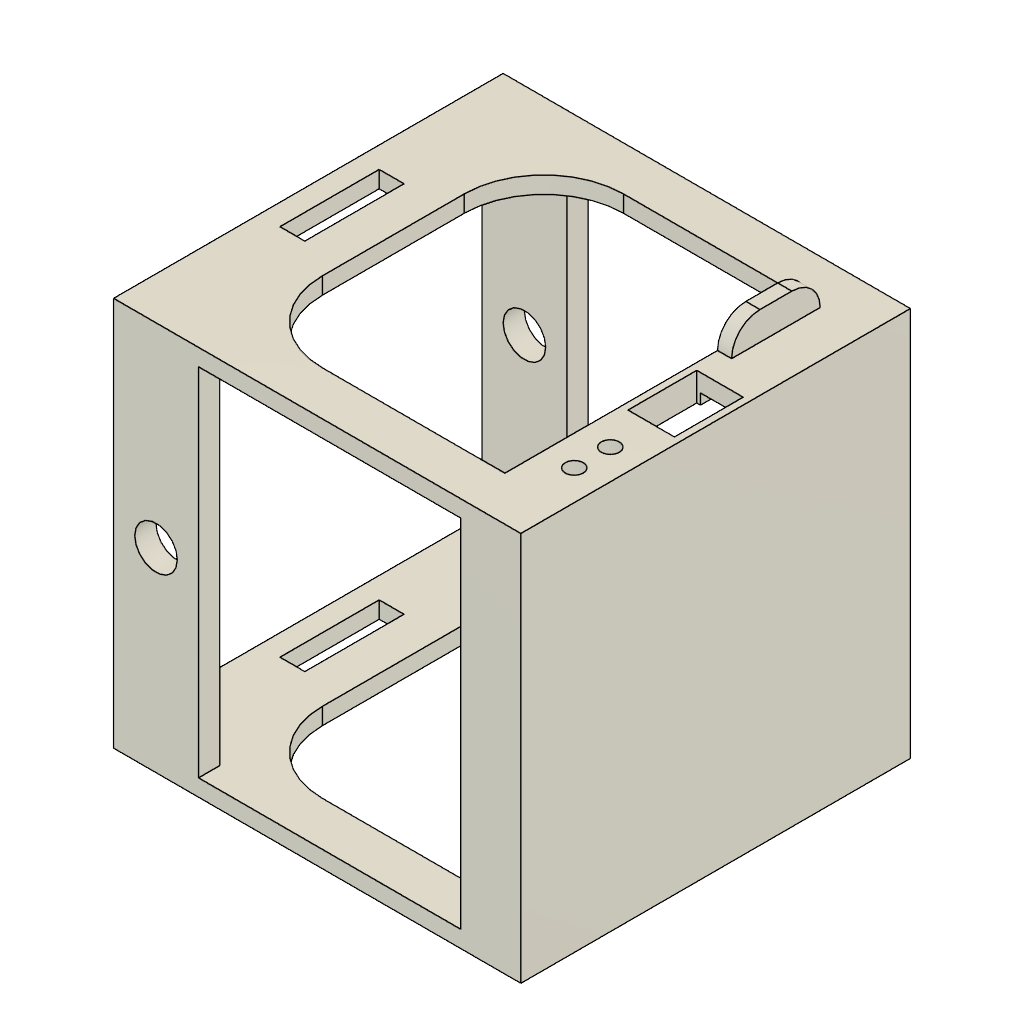
Cansat_D1 (Autodesk Fusion 360 design; units mm, degrees)
part number: 2026-09-08-22-36-42-588
Autodesk Fusion 360 part; units mm, degrees
note: some values were not read from the file. Set by a fixed rule: which sketch regions a step uses.
sketch "Sketch1" plane through (0, 0, 0) normal (0, 1, 0) x (1, 0, 0)
  line L0 (-55, -55) -> (55, -55)
  line L1 (55, -55) -> (55, 55)
  line L2 (55, 55) -> (-55, 55)
  line L3 (-55, 55) -> (-55, -55)
  line L4 (-55, -55) -> (55, 55) construction
  line L5 (55, -55) -> (-55, 55) construction
  line L6 (-50, 50) -> (50, 50)
  line L7 (50, 50) -> (50, -50)
  line L8 (50, -50) -> (-50, -50)
  line L9 (-50, -50) -> (-50, 50)
  line L10 (-50, 50) -> (50, -50) construction
  line L11 (50, 50) -> (-50, -50) construction
  dimension "d1" = 110
  dimension "d2" = 110
  dimension "d3" = 100
  dimension "d4" = 100
  constraint horizontal L0
  constraint perpendicular L0 L1
  constraint parallel L0 L2
  constraint parallel L1 L3
  constraint coincident L4 origin
  constraint coincident L5 origin
  constraint horizontal L6
  constraint perpendicular L6 L7
  constraint parallel L6 L8
  constraint parallel L7 L9
  constraint coincident L10 origin
  constraint coincident L11 origin
  measures "d1" distance of L1.end L2.end
  measures "d2" distance of L0.end L1.end
  measures "d3" distance of L7.end L8.end
  measures "d4" distance of L6.end L7.end
extrude "Extrude1" add sketch "Sketch1" along normal blind 5 contours L6 L7 L8 L9 makes body 1
extrude "Extrude2" add sketch "Sketch1" along normal blind 15 bodies 1
extrude "Extrude3" cut 1 faces at (-16.6667, 5, -16.6667) along direction (0, -1, 0) blind 1 on bodies 1 bodies 1
sketch "Sketch2" plane through (0, 15, 0) normal (0, 1, 0) x (-1, 0, 0)
  line L0 (-50, 50) -> (50, 50)
  line L1 (50, 50) -> (50, -50)
  line L2 (50, -50) -> (-50, -50)
  line L3 (-50, -50) -> (-50, 50)
  line L4 (55, -55) -> (55, 55)
  line L5 (55, 55) -> (-55, 55)
  line L6 (-55, 55) -> (-55, -55)
  line L7 (-55, -55) -> (55, -55)
sketch "Sketch3" plane through (0, 15, 0) normal (0, 1, 0) x (-1, 0, 0)
  line L0 (55, -55) -> (50, -55)
  line L1 (50, -55) -> (50, 55)
  line L2 (50, 55) -> (55, 55)
  line L3 (55, 55) -> (55, -55)
  line L4 (-50, -55) -> (-55, -55)
  line L5 (-55, -55) -> (-55, 55)
  line L6 (-55, 55) -> (-50, 55)
  line L7 (-50, 55) -> (-50, -55)
  constraint horizontal L0
  constraint vertical L1
  constraint horizontal L2
  constraint vertical L3
  constraint horizontal L4
  constraint vertical L5
  constraint horizontal L6
  constraint vertical L7
extrude "Extrude4" add sketch "Sketch3" along normal blind 100 bodies 1
sketch "Sketch4" plane through (55, 0, 0) normal (1, 0, 0) x (0, 0, -1)
  line L0 (-55, 0) -> (55, 0)
  line L1 (55, 0) -> (55, 115)
  line L2 (55, 115) -> (-55, 115)
  line L3 (-55, 115) -> (-55, 0)
  line L4 (0, 115) -> (0, 109)
  line L5 (0, 109) -> (0, 102)
  line L6 (0, 102) -> (0, 105.5)
  line L7 (0, 105.5) -> (55, 105.5)
  line L8 (55, 105.5) -> (49, 105.5)
  line L9 (49, 109) -> (-49, 109)
  line L10 (-49, 109) -> (-49, 102)
  line L11 (-49, 102) -> (49, 102)
  line L12 (49, 102) -> (49, 109)
  line L13 (49, 109) -> (-49, 102) construction
  line L14 (-49, 109) -> (49, 102) construction
  point P0 (0, 105.5)
  dimension "d13" = 98
  dimension "d14" = 7
  constraint midpoint L2 L4.start
  constraint perpendicular L2 L4
  constraint perpendicular L2 L5
  constraint midpoint L5 P0
  constraint coincident L1 L7.end
  constraint perpendicular L1 L7
  constraint coincident L7 L8.end
  constraint horizontal L9
  constraint perpendicular L9 L10
  constraint parallel L9 L11
  constraint parallel L10 L12
  constraint coincident L13 P0
  constraint coincident L14 P0
  constraint coincident P0 L6.end
  measures "d13" distance of L10.end L11.end
  measures "d14" distance of L9.end L10.end
extrude "Extrude5" cut sketch "Sketch4" against normal blind 163 contours L5 L6 L7 L11 L12 | L5 L7 L9 L12 | L5 L6 L9 L10 L11 bodies 1
sketch "Sketch5" plane through (55, 0, 0) normal (1, 0, 0) x (0, 0, -1)
  line L0 (-49, 109) -> (49, 109)
  line L1 (49, 109) -> (49, 102)
  line L2 (49, 102) -> (-49, 102)
  line L3 (-49, 102) -> (-49, 109)
  line L4 (-55, 0) -> (55, 0)
  line L5 (55, 0) -> (55, 115)
  line L6 (55, 115) -> (-55, 115)
  line L7 (-55, 115) -> (-55, 0)
  line L8 (-55, 115) -> (-49, 115)
  line L9 (-49, 115) -> (-49, 109)
  line L10 (-49, 109) -> (-55, 109)
  line L11 (-55, 109) -> (-55, 115)
  line L12 (55, 115) -> (49, 115)
  line L13 (49, 115) -> (49, 109)
  line L14 (49, 109) -> (55, 109)
  line L15 (55, 109) -> (55, 115)
  constraint horizontal L8
  constraint vertical L9
  constraint horizontal L10
  constraint vertical L11
  constraint coincident L0.start L3.end
  constraint coincident L6.end L7.start
  constraint horizontal L12
  constraint vertical L13
  constraint horizontal L14
  constraint vertical L15
  constraint coincident L0.end L1.start
  constraint coincident L5.end L6.start
extrude "Extrude6" add sketch "Sketch5" against normal blind 110 separate body contours L6 L7 L8 L9 L10 L11 | L5 L6 L12 L13 L14 L15 makes body 2 at (18.3333, 109, 51) makes body 3 at (18.3333, 115, -53)
sketch "Sketch6" plane through (55, 0, 0) normal (1, 0, 0) x (0, 0, -1)
  line L0 (-49, 109) -> (49, 109)
  line L1 (49, 109) -> (49, 102)
  line L2 (49, 102) -> (-49, 102)
  line L3 (-49, 102) -> (-49, 109)
  line L4 (-55, 0) -> (55, 0)
  line L5 (55, 0) -> (55, 115)
  line L6 (55, 115) -> (-55, 115)
  line L7 (-55, 115) -> (-55, 0)
  line L8 (0, 102) -> (0, 58.5)
  line L9 (32.5, 91) -> (-32.5, 91)
  line L10 (-32.5, 91) -> (-32.5, 26)
  line L11 (-32.5, 26) -> (32.5, 26)
  line L12 (32.5, 26) -> (32.5, 91)
  line L13 (32.5, 91) -> (-32.5, 26) construction
  line L14 (-32.5, 91) -> (32.5, 26) construction
  point P0 (0, 58.5)
  dimension "d19" = 43.5
  dimension "d20" = 65
  dimension "d21" = 65
  constraint vertical L8
  constraint midpoint L2 L8.start
  constraint horizontal L9
  constraint perpendicular L9 L10
  constraint parallel L9 L11
  constraint parallel L10 L12
  constraint coincident L13 P0
  constraint coincident L14 P0
  constraint coincident P0 L8.end
  measures "d19" distance of L8.start P0
  measures "d20" distance of L10.end L11.end
  measures "d21" distance of L9.end L10.end
extrude "Extrude7" cut sketch "Sketch6" against normal blind 435 contours L9 L10 L11 L12 bodies 1
extrude "Extrude8" add 2 faces at (18.3333, 109, -51) (18.3333, 109, 51) along direction (0, -1, 0) blind 7 on bodies 2 3 bodies 1 3 2
extrude "Extrude9" cut 2 faces at (-51.6667, 26, 10.8333) (51.6667, 26, 10.8333) along direction (0, -1, 0) blind 11 on bodies 1 bodies 1
extrude "Extrude10" cut 2 faces at (53.3333, 65.6667, 32.5) (-51.6667, 65.6667, 32.5) along direction (0, 0, 1) blind 10 on bodies 1 bodies 1
extrude "Extrude11" cut 2 faces at (53.3333, 40.3333, -32.5) (-51.6667, 40.3333, -32.5) along direction (0, 0, -1) blind 10 on bodies 1 bodies 1
extrude "Extrude13" add 2 faces at (-16.6667, 102, 51) (-16.6667, 102, -51) along direction (0, -1, 0) blind 11 on bodies 1 bodies 1
fillet "Fillet2" radius 22.5 4 edges at (-52.5, 91, -42.5) (-52.5, 91, 42.5) (52.5, 91, 42.5) (52.5, 91, -42.5) on bodies 1
move_body "Move1" bodies 1 to x (0, 1, 0) y (-1, 0, 0) z (0, 0, 1) at (52.7274, 53.5, -21.0589)
move_body "Move2" bodies 1 to x (1, 0, 0) y (0, 1, 0) z (0, 0, 1) at (0, 2, 0)
extrude "Extrude14" add 4 faces at (37.7274, 72.1667, 32.2744) (37.7274, 108.8333, -6.8923) (37.7274, 38.8333, -74.3923) (37.7274, 3.8333, -35.2256) along direction (-1, 0, 0) blind 2 on bodies 1 bodies 1
sketch "Sketch8" plane through (0, 0, -76.0589) normal (0, 0, -1) x (-1, 0, 0)
  line L0 (-35.7274, 105.5) -> (38.2726, 105.5)
  line L1 (38.2726, 105.5) -> (38.2726, 5.5)
  line L2 (38.2726, 5.5) -> (-35.7274, 5.5)
  line L3 (-35.7274, 5.5) -> (-35.7274, 105.5)
  line L4 (-52.7274, 0.5) -> (62.2726, 0.5)
  line L5 (62.2726, 0.5) -> (62.2726, 110.5)
  line L6 (62.2726, 110.5) -> (-52.7274, 110.5)
  line L7 (-52.7274, 110.5) -> (-52.7274, 0.5)
  line L8 (-35.7274, 105.5) -> (-38.7274, 105.5)
  line L9 (-38.7274, 105.5) -> (-38.7274, 5.5)
  line L10 (-38.7274, 5.5) -> (-35.7274, 5.5)
  line L11 (-35.7274, 5.5) -> (-35.7274, 105.5)
  dimension "d44" = 3
  dimension "d45" = 100
  constraint horizontal L8
  constraint vertical L9
  constraint horizontal L10
  constraint vertical L11
  constraint coincident L0.start L3.end
  measures "d44" distance of L0.start L8.end
  measures "d45" distance of L0.start L2.end
sketch "Sketch9" plane through (0, 110.5, 0) normal (0, 1, 0) x (-1, 0, 0)
  line L0 (-35.7274, -63.5589) -> (-35.7274, 21.4411)
  line L1 (-35.7274, 21.4411) -> (15.7726, 21.4411)
  arc A0 (38.2726, -1.0589) -> (15.7726, 21.4411) centre (15.7726, -1.0589) ccw
  line L2 (38.2726, -1.0589) -> (38.2726, -41.0589)
  arc A1 (15.7726, -63.5589) -> (38.2726, -41.0589) centre (15.7726, -41.0589) ccw
  line L3 (15.7726, -63.5589) -> (-35.7274, -63.5589)
  line L4 (62.2726, 33.9411) -> (-52.7274, 33.9411)
  line L5 (-52.7274, 33.9411) -> (-52.7274, -76.0589)
  line L6 (-52.7274, -76.0589) -> (62.2726, -76.0589)
  line L7 (62.2726, -76.0589) -> (62.2726, 33.9411)
  line L8 (49.2726, 27.9411) -> (56.2726, 27.9411)
  line L9 (56.2726, 27.9411) -> (56.2726, -70.0589)
  line L10 (56.2726, -70.0589) -> (49.2726, -70.0589)
  line L11 (49.2726, -70.0589) -> (49.2726, 27.9411)
  line L12 (-35.7274, 21.4411) -> (-38.7274, 21.4411)
  line L13 (-38.7274, 21.4411) -> (-38.7274, -63.5589)
  line L14 (-38.7274, -63.5589) -> (-35.7274, -63.5589)
  line L15 (-35.7274, -63.5589) -> (-35.7274, 21.4411)
  dimension "d46" = 3
  dimension "d47" = 85
  constraint horizontal L12
  constraint vertical L13
  constraint horizontal L14
  constraint vertical L15
  constraint coincident L0.end L1.start
  measures "d46" distance of L0.end L12.end
  measures "d47" distance of L0.end L0.start
sketch "Sketch10" plane through (0, 0.5, 0) normal (0, -1, 0) x (1, 0, 0)
  line L0 (-38.2726, -41.0589) -> (-38.2726, -1.0589)
  arc A0 (-15.7726, 21.4411) -> (-38.2726, -1.0589) centre (-15.7726, -1.0589) ccw
  line L1 (-15.7726, 21.4411) -> (35.7274, 21.4411)
  line L2 (35.7274, 21.4411) -> (35.7274, -63.5589)
  line L3 (35.7274, -63.5589) -> (-15.7726, -63.5589)
  arc A1 (-38.2726, -41.0589) -> (-15.7726, -63.5589) centre (-15.7726, -41.0589) ccw
  line L4 (-49.2726, 27.9411) -> (-49.2726, -70.0589)
  line L5 (-49.2726, -70.0589) -> (-56.2726, -70.0589)
  line L6 (-56.2726, -70.0589) -> (-56.2726, 27.9411)
  line L7 (-56.2726, 27.9411) -> (-49.2726, 27.9411)
  line L8 (52.7274, 33.9411) -> (-62.2726, 33.9411)
  line L9 (-62.2726, 33.9411) -> (-62.2726, -76.0589)
  line L10 (-62.2726, -76.0589) -> (52.7274, -76.0589)
  line L11 (52.7274, -76.0589) -> (52.7274, 33.9411)
  line L12 (35.7274, -63.5589) -> (38.7274, -63.5589)
  line L13 (38.7274, -63.5589) -> (38.7274, 21.4411)
  line L14 (38.7274, 21.4411) -> (35.7274, 21.4411)
  line L15 (35.7274, 21.4411) -> (35.7274, -63.5589)
  dimension "d48" = 3
  dimension "d49" = 85
  constraint horizontal L12
  constraint vertical L13
  constraint horizontal L14
  constraint vertical L15
  constraint coincident L2.end L3.start
  measures "d48" distance of L2.end L12.end
  measures "d49" distance of L2.end L1.end
sketch "Sketch11" plane through (0, 0, 33.9411) normal (0, 0, 1) x (1, 0, 0)
  line L0 (-62.2726, 0.5) -> (52.7274, 0.5)
  line L1 (52.7274, 0.5) -> (52.7274, 110.5)
  line L2 (52.7274, 110.5) -> (-62.2726, 110.5)
  line L3 (-62.2726, 110.5) -> (-62.2726, 0.5)
  line L4 (35.7274, 105.5) -> (35.7274, 5.5)
  line L5 (35.7274, 5.5) -> (-38.2726, 5.5)
  line L6 (-38.2726, 5.5) -> (-38.2726, 105.5)
  line L7 (-38.2726, 105.5) -> (35.7274, 105.5)
  line L8 (35.7274, 5.5) -> (38.7274, 5.5)
  line L9 (38.7274, 5.5) -> (38.7274, 105.5)
  line L10 (38.7274, 105.5) -> (35.7274, 105.5)
  line L11 (35.7274, 105.5) -> (35.7274, 5.5)
  dimension "d50" = 3
  dimension "d51" = 100
  constraint horizontal L8
  constraint vertical L9
  constraint horizontal L10
  constraint vertical L11
  constraint coincident L4.end L5.start
  measures "d50" distance of L4.end L8.end
  measures "d51" distance of L4.end L4.start
extrude "Extrude15" add sketch "Sketch10" against normal blind 8 contours L2 L12 L13 L14 L15 bodies 1
extrude "Extrude16" add sketch "Sketch11" against normal blind 8 separate body contours L4 L8 L9 L10 L11 makes body 4
extrude "Extrude17" add 1 faces at (37.3941, 7.5, 21.4411) along direction (0, 0, 1) blind 5 on bodies 1 bodies 1 4
extrude "Extrude18" add sketch "Sketch9" against normal blind 8 separate body contours L0 L12 L13 L14 L15 makes body 5
extrude "Extrude19" add 1 faces at (36.7274, 107.8333, 21.4411) along direction (0, 0, 1) blind 5 on bodies 5 bodies 1 5
extrude "Extrude20" cut sketch "Sketch8" against normal blind 5 contours L3 L8 L9 L10 L11 bodies 1
extrude "Extrude21" add 2 faces at (37.3941, 7.5, -63.5589) (37.7274, 104.5, -63.5589) along direction (0, 0, -1) blind 12.5 on bodies 1 bodies 1
sketch "Sketch12" plane through (0, 0, -70.0589) normal (0, 0, 1) x (1, 0, 0)
  line L0 (-56.2726, 5.5) -> (-56.2726, 0.5)
  line L1 (-56.2726, 0.5) -> (-49.2726, 0.5)
  line L2 (-49.2726, 0.5) -> (-49.2726, 5.5)
  line L3 (-49.2726, 5.5) -> (-38.2726, 5.5)
  line L4 (-38.2726, 5.5) -> (-38.2726, 105.5)
  line L5 (-38.2726, 105.5) -> (-49.2726, 105.5)
  line L6 (-49.2726, 105.5) -> (-49.2726, 110.5)
  line L7 (-49.2726, 110.5) -> (-56.2726, 110.5)
  line L8 (-56.2726, 110.5) -> (-56.2726, 105.5)
  line L9 (-56.2726, 105.5) -> (-62.2726, 105.5)
  line L10 (-62.2726, 105.5) -> (-62.2726, 5.5)
  line L11 (-62.2726, 5.5) -> (-56.2726, 5.5)
  line L12 (-56.2726, 110.5) -> (-49.2726, 110.5)
  line L13 (-49.2726, 110.5) -> (-49.2726, 105.5)
  line L14 (-49.2726, 105.5) -> (-56.2726, 105.5)
  line L15 (-56.2726, 105.5) -> (-56.2726, 110.5)
  line L16 (-56.2726, 5.5) -> (-49.2726, 5.5)
  line L17 (-49.2726, 5.5) -> (-49.2726, 0.5)
  line L18 (-49.2726, 0.5) -> (-56.2726, 0.5)
  line L19 (-56.2726, 0.5) -> (-56.2726, 5.5)
  constraint horizontal L12
  constraint vertical L13
  constraint horizontal L14
  constraint vertical L15
  constraint coincident L5.end L6.start
  constraint coincident L7.end L8.start
  constraint horizontal L16
  constraint vertical L17
  constraint horizontal L18
  constraint vertical L19
  constraint coincident L1.end L2.start
  constraint coincident L0.start L11.end
extrude "Extrude22" add sketch "Sketch12" along normal blind 30 contours L0 L1 L2 L16 L17 L18 L19 | L6 L7 L8 L12 L13 L14 L15 bodies 1
sketch "Sketch13" plane through (0, 0, 27.9411) normal (0, 0, -1) x (-1, 0, 0)
  line L0 (49.2726, 5.5) -> (49.2726, 0.5)
  line L1 (49.2726, 0.5) -> (56.2726, 0.5)
  line L2 (56.2726, 0.5) -> (56.2726, 5.5)
  line L3 (56.2726, 5.5) -> (62.2726, 5.5)
  line L4 (62.2726, 5.5) -> (62.2726, 105.5)
  line L5 (62.2726, 105.5) -> (56.2726, 105.5)
  line L6 (56.2726, 105.5) -> (56.2726, 110.5)
  line L7 (56.2726, 110.5) -> (49.2726, 110.5)
  line L8 (49.2726, 110.5) -> (49.2726, 105.5)
  line L9 (49.2726, 105.5) -> (38.2726, 105.5)
  line L10 (38.2726, 105.5) -> (38.2726, 5.5)
  line L11 (38.2726, 5.5) -> (49.2726, 5.5)
  line L12 (49.2726, 110.5) -> (56.2726, 110.5)
  line L13 (56.2726, 110.5) -> (56.2726, 105.5)
  line L14 (56.2726, 105.5) -> (49.2726, 105.5)
  line L15 (49.2726, 105.5) -> (49.2726, 110.5)
  line L16 (49.2726, 5.5) -> (56.2726, 5.5)
  line L17 (56.2726, 5.5) -> (56.2726, 0.5)
  line L18 (56.2726, 0.5) -> (49.2726, 0.5)
  line L19 (49.2726, 0.5) -> (49.2726, 5.5)
  constraint horizontal L12
  constraint vertical L13
  constraint horizontal L14
  constraint vertical L15
  constraint coincident L5.end L6.start
  constraint coincident L7.end L8.start
  constraint horizontal L16
  constraint vertical L17
  constraint horizontal L18
  constraint vertical L19
  constraint coincident L1.end L2.start
  constraint coincident L0.start L11.end
extrude "Extrude23" add sketch "Sketch13" along normal blind 35 contours L0 L1 L2 L16 L17 L18 L19 | L6 L7 L8 L12 L13 L14 L15 bodies 1
extrude "Extrude24" add 2 faces at (-53.9393, 3.8333, -40.0589) (-51.6059, 108.8333, -40.0589) along direction (0, 0, 1) blind 5 on bodies 1 bodies 1
sketch "Sketch14" plane through (0, 0, -76.0589) normal (0, 0, -1) x (-1, 0, 0)
  line L0 (-35.7274, 105.5) -> (38.2726, 105.5)
  line L1 (38.2726, 105.5) -> (38.2726, 5.5)
  line L2 (38.2726, 5.5) -> (-35.7274, 5.5)
  line L3 (-35.7274, 5.5) -> (-35.7274, 8.5)
  line L4 (-35.7274, 8.5) -> (-38.7274, 8.5)
  line L5 (-38.7274, 8.5) -> (-38.7274, 102.5)
  line L6 (-38.7274, 102.5) -> (-35.7274, 102.5)
  line L7 (-35.7274, 102.5) -> (-35.7274, 105.5)
  line L8 (-52.7274, 0.5) -> (62.2726, 0.5)
  line L9 (62.2726, 0.5) -> (62.2726, 110.5)
  line L10 (62.2726, 110.5) -> (-52.7274, 110.5)
  line L11 (-52.7274, 110.5) -> (-52.7274, 0.5)
  line L12 (62.2726, 110.5) -> (38.2726, 110.5)
  line L13 (38.2726, 110.5) -> (38.2726, 0.5)
  line L14 (38.2726, 0.5) -> (62.2726, 0.5)
  line L15 (62.2726, 0.5) -> (62.2726, 110.5)
  line L16 (50.2726, 110.5) -> (50.2726, 0.5)
  line L17 (38.2726, 55.5) -> (62.2726, 55.5)
  circle A0 centre (50.2726, 55.5) radius 6
  dimension "d72" = 12
  constraint horizontal L12
  constraint vertical L13
  constraint horizontal L14
  constraint vertical L15
  constraint coincident L8 L13.end
  constraint coincident L9.end L10.start
  constraint midpoint L12 L16.start
  constraint midpoint L14 L16.end
  constraint midpoint L13 L17.start
  constraint midpoint L9 L17.end
  constraint midpoint L16 A0.centre
  measures "d72" diameter of A0
extrude "Extrude25" cut sketch "Sketch14" against normal blind 400 contours L16 L17 A0 | L16 L17 A0 | L16 L17 A0 | L16 L17 A0 bodies 1
extrude "Extrude26" cut 1 faces at (-49.9688, 5.5, 8.7207) along direction (0, -1, 0) blind 0.25 on bodies 1 bodies 1
extrude "Extrude27" cut 1 faces at (-51.9688, 105.5, 8.7207) along direction (0, 1, 0) blind 0.25 on bodies 1 bodies 1
sketch "Sketch15" plane through (0, 110.5, 0) normal (0, 1, 0) x (-1, 0, 0)
  line L0 (-35.7274, 21.4411) -> (15.7726, 21.4411)
  arc A0 (38.2726, -1.0589) -> (15.7726, 21.4411) centre (15.7726, -1.0589) ccw
  line L1 (38.2726, -1.0589) -> (38.2726, -41.0589)
  arc A1 (15.7726, -63.5589) -> (38.2726, -41.0589) centre (15.7726, -41.0589) ccw
  line L2 (15.7726, -63.5589) -> (-35.7274, -63.5589)
  line L3 (-35.7274, -63.5589) -> (-35.7274, 21.4411)
  line L4 (62.2726, 33.9411) -> (-52.7274, 33.9411)
  line L5 (-52.7274, 33.9411) -> (-52.7274, -76.0589)
  line L6 (-52.7274, -76.0589) -> (62.2726, -76.0589)
  line L7 (62.2726, -76.0589) -> (62.2726, 33.9411)
  line L8 (49.2726, -7.0589) -> (56.2726, -7.0589)
  line L9 (56.2726, -7.0589) -> (56.2726, -35.0589)
  line L10 (56.2726, -35.0589) -> (49.2726, -35.0589)
  line L11 (49.2726, -35.0589) -> (49.2726, -7.0589)
  line L12 (-35.7274, -63.5589) -> (-39.7274, -63.5589)
  line L13 (-52.7274, 21.4411) -> (-35.7274, 21.4411)
  line L14 (-35.7274, -38.5589) -> (-35.7274, -63.5589)
  line L15 (-35.7274, -63.5589) -> (-39.7274, -63.5589)
  line L16 (-39.7274, -63.5589) -> (-39.7274, -38.5589)
  line L17 (-39.7274, -38.5589) -> (-35.7274, -38.5589)
  line L18 (-35.7274, -38.5589) -> (-35.7274, -63.5589)
  dimension "d79" = 4
  dimension "d80" = 25
  constraint horizontal L12
  constraint horizontal L13
  constraint vertical L14
  constraint coincident L5 L13.start
  constraint coincident L2.end L3.start
  constraint horizontal L15
  constraint vertical L16
  constraint horizontal L17
  constraint vertical L18
  measures "d79" distance of L2.end L12.end
  measures "d80" distance of L2.end L14.start
extrude "Extrude28" add sketch "Sketch15" along normal blind 8 contours L3 L12 L14 L15 L16 L17 L18 bodies 1
fillet "Fillet3" radius 8 2 edges at (37.7274, 118.5, -38.5589) (37.7274, 118.5, -63.5589) on bodies 1
sketch "Sketch16" plane through (0, 110.5, 0) normal (0, 1, 0) x (-1, 0, 0)
  line L0 (49.2726, -7.0589) -> (56.2726, -7.0589)
  line L1 (56.2726, -7.0589) -> (56.2726, -35.0589)
  line L2 (56.2726, -35.0589) -> (49.2726, -35.0589)
  line L3 (49.2726, -35.0589) -> (49.2726, -7.0589)
  line L4 (62.2726, 33.9411) -> (-52.7274, 33.9411)
  line L5 (-52.7274, 33.9411) -> (-52.7274, -76.0589)
  line L6 (-52.7274, -76.0589) -> (62.2726, -76.0589)
  line L7 (62.2726, -76.0589) -> (62.2726, 33.9411)
  line L8 (-35.7274, -63.5589) -> (-39.7274, -63.5589)
  line L9 (-39.7274, -63.5589) -> (-39.7274, -38.5589)
  line L10 (-39.7274, -38.5589) -> (-35.7274, -38.5589)
  line L11 (-35.7274, -38.5589) -> (-35.7274, 21.4411)
  line L12 (-35.7274, 21.4411) -> (15.7726, 21.4411)
  arc A0 (38.2726, -1.0589) -> (15.7726, 21.4411) centre (15.7726, -1.0589) ccw
  line L13 (38.2726, -1.0589) -> (38.2726, -41.0589)
  arc A1 (15.7726, -63.5589) -> (38.2726, -41.0589) centre (15.7726, -41.0589) ccw
  line L14 (15.7726, -63.5589) -> (-35.7274, -63.5589)
  line L15 (-35.7274, 21.4411) -> (-52.7274, 21.4411)
  line L16 (-35.7274, -63.5589) -> (-52.7274, -63.5589)
  line L17 (-52.7274, -63.5589) -> (-35.7274, 21.4411)
  line L18 (-52.7274, 21.4411) -> (-35.7274, -63.5589)
  line L19 (-44.2274, -21.0589) -> (-35.7274, -21.0589)
  line L20 (-37.6774, -30.7589) -> (-50.7774, -30.7589)
  line L21 (-50.7774, -30.7589) -> (-50.7774, -11.3589)
  line L22 (-50.7774, -11.3589) -> (-37.6774, -11.3589)
  line L23 (-37.6774, -11.3589) -> (-37.6774, -30.7589)
  line L24 (-37.6774, -30.7589) -> (-50.7774, -11.3589) construction
  line L25 (-50.7774, -30.7589) -> (-37.6774, -11.3589) construction
  line L26 (-44.2274, -21.0589) -> (-44.2274, 21.4411)
  circle A2 centre (-44.2274, 0.1911) radius 2.55
  circle A3 centre (-44.2274, 10.3629) radius 2.55
  point P0 (-44.2274, -21.0589)
  dimension "d85" = 13.1
  dimension "d86" = 19.4
  dimension "d89" = 5.1
  dimension "d90" = 5.1
  constraint coincident L11.end L12.start
  constraint coincident L5 L15.end
  constraint perpendicular L5 L15
  constraint coincident L8.start L14.end
  constraint coincident L5 L16.end
  constraint perpendicular L5 L16
  constraint midpoint L17 P0
  constraint coincident L11 L19.end
  constraint perpendicular L11 L19
  constraint horizontal L20
  constraint perpendicular L20 L21
  constraint parallel L20 L22
  constraint parallel L21 L23
  constraint coincident L24 P0
  constraint coincident L25 P0
  constraint coincident P0 L19.start
  constraint midpoint L15 L26.end
  constraint midpoint L26 A2.centre
  constraint coincident L26 A3.centre
  measures "d85" distance of L21.end L22.end
  measures "d86" distance of L20.end L21.end
  measures "d89" diameter of A2
  measures "d90" diameter of A3
extrude "Extrude29" cut sketch "Sketch16" against normal blind 10 contours L18 L22 L26 | L17 L18 L20 L21 L22 | L17 L18 L20 | L17 L22 L26 | L18 L19 L20 L23 | L17 L19 L22 L23 bodies 1
extrude "Extrude30" cut sketch "Sketch16" against normal blind 13 contours L26 A3 | L26 A3 | L26 A2 | L26 A2 bodies 1
equation "d19 = ( 87 / 2 ) * 1 mm"
